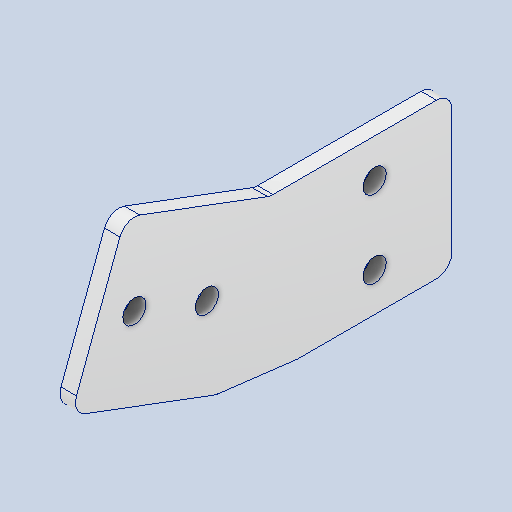
# Autodesk Inventor part: RZvector-v1-MP-Tr-F
Saved by Autodesk Inventor 2025.1 (Build 291241000, 241)
## iProperties
Created: 2024-03-17
Part Number: RZvector-v1-MP-Tr-F
Material: アルミニウム 6061
Document SubType Name: Modeling
Designer: haruy
Density: 2.7 g/cm^3
Appearance: アルミニウム - フラット
Mass: 1.7478 g
Surface Area: 21.5742 cm^2
Volume: 2.18475 cm^3
Author: haruy
Autodesk Inventor part; units mm, degrees
ref_plane "YZ Plane" through (0, 0, 0) normal (1, 0, 0) x (0, 1, 0)
ref_plane "XZ Plane" through (0, 0, 0) normal (0, 1, 0) x (-1, 0, 0)
ref_plane "XY Plane" through (0, 0, 0) normal (0, 0, 1) x (1, 0, 0)
derived "RZvector-arm-rotate-v1-Sketch-Base.ipt"
sketch "横から" plane through (0, 0, 0) normal (1, 0, 0) x (0, 1, 0)
  line L0 (0, 0) -> (0, -30.2937)
  line L1 (542.7807, -196.25) -> (0, -196.25)
  line L2 (628, -186.25) -> (24, -186.25)
  line L3 (24, -186.25) -> (24, -206.25)
  line L4 (24, -206.25) -> (628, -206.25)
  line L5 (628, -206.25) -> (628, -186.25)
  line L6 (138, -159.75) -> (123, -159.75)
  line L7 (123, -159.75) -> (123, -174.75)
  line L8 (123, -174.75) -> (138, -174.75)
  line L9 (138, -174.75) -> (138, -159.75)
  line L10 (0, 0) -> (0, -196.25)
  line L11 (138, -217.75) -> (123, -217.75)
  line L12 (123, -217.75) -> (123, -232.75)
  line L13 (123, -232.75) -> (138, -232.75)
  line L14 (138, -232.75) -> (138, -217.75)
  line L15 (0, 0) -> (0, -415.25)
  line L16 (54, -415.25) -> (34, -415.25)
  line L17 (34, -415.25) -> (34, -395.25)
  line L18 (34, -395.25) -> (54, -395.25)
  line L19 (54, -395.25) -> (54, -415.25)
  line L20 (134, -345.25) -> (64, -345.25)
  line L21 (64, -345.25) -> (64, -395.25)
  line L22 (64, -395.25) -> (134, -395.25)
  line L23 (134, -395.25) -> (134, -345.25)
  line L24 (136, -310.25) -> (134, -310.25)
  line L25 (134, -310.25) -> (134, -405.25)
  line L26 (134, -405.25) -> (136, -405.25)
  line L27 (136, -405.25) -> (136, -310.25)
  line L28 (136, -310.25) -> (146, -310.25)
  line L29 (146, -310.25) -> (146, -320.25)
  line L30 (146, -320.25) -> (136, -320.25)
  line L31 (136, -320.25) -> (136, -310.25)
  line L32 (146, -320.25) -> (54, -320.25)
  line L33 (54, -320.25) -> (54, -330.25)
  line L34 (54, -330.25) -> (146, -330.25)
  line L35 (146, -330.25) -> (146, -320.25)
  line L36 (0, -269) -> (385.3867, -269)
  line L37 (144, 54.75) -> (46, 54.75)
  line L38 (46, 54.75) -> (46, -139.45)
  line L39 (46, -139.45) -> (144, -139.45)
  line L40 (144, -139.45) -> (144, 54.75)
  circle A0 centre (95, 2.25) radius 95
  line L41 (176, -92.75) -> (156, -92.75)
  line L42 (156, -92.75) -> (156, -290.75)
  line L43 (156, -290.75) -> (176, -290.75)
  line L44 (176, -290.75) -> (176, -92.75)
  circle A1 centre (166, -269) radius 6
  circle A2 centre (166, -269) radius 22.5
  circle A3 centre (129.5351, -260.25) radius 15
  circle A4 centre (129.5351, -260.25) radius 6
  line L45 (138, -159.75) -> (153, -159.75)
  line L46 (153, -159.75) -> (153, -232.75)
  line L47 (153, -232.75) -> (138, -232.75)
  line L48 (138, -232.75) -> (138, -159.75)
  line L49 (123, -174.75) -> (153, -174.75)
  line L50 (153, -174.75) -> (153, -184.75)
  line L51 (153, -184.75) -> (123, -184.75)
  line L52 (123, -184.75) -> (123, -174.75)
  line L53 (123, -217.75) -> (153, -217.75)
  line L54 (153, -217.75) -> (153, -207.75)
  line L55 (153, -207.75) -> (123, -207.75)
  line L56 (123, -207.75) -> (123, -217.75)
  circle A5 centre (129.5351, -260.25) radius 18.75
  circle A6 centre (99.5351, -260.25) radius 15
  line L57 (136, -330.25) -> (146, -330.25)
  line L58 (146, -330.25) -> (146, -340.25)
  line L59 (146, -340.25) -> (136, -340.25)
  line L60 (136, -340.25) -> (136, -330.25)
  line L61 (54, -405.25) -> (56, -405.25)
  line L62 (56, -405.25) -> (56, -345.2512)
  line L63 (56, -345.2512) -> (54, -345.2512)
  line L64 (54, -345.2512) -> (54, -405.25)
  line L65 (56, -320.25) -> (64.683, -320.25)
  line L66 (54, -310.25) -> (64, -310.25)
  line L67 (64, -310.25) -> (64, -320.25)
  line L68 (64, -320.25) -> (54, -320.25)
  line L69 (54, -320.25) -> (54, -310.25)
  line L70 (54, -310.25) -> (44, -310.25)
  line L71 (44, -310.25) -> (44, -340.25)
  line L72 (44, -340.25) -> (54, -340.25)
  line L73 (54, -340.25) -> (54, -310.25)
  line L74 (34, -415.25) -> (54, -415.25)
  line L75 (54, -415.25) -> (54, -139.45)
  line L76 (54, -139.45) -> (34, -139.45)
  line L77 (34, -139.45) -> (34, -415.25)
  line L78 (628, -186.25) -> (659.5, -186.25)
  line L79 (659.5, -186.25) -> (659.5, -206.25)
  line L80 (659.5, -206.25) -> (628, -206.25)
  line L81 (628, -206.25) -> (628, -186.25)
  line L82 (54, -375.25) -> (34, -375.25)
  circle A7 centre (129.5351, -260.25) radius 12.5
  circle A8 centre (643.75, -167.5) radius 15.75
  line L83 (659.5, -186.25) -> (659.5, -167.5)
  line L84 (628, -186.25) -> (628, -167.5)
  line L85 (150.5, -293.5212) -> (150.5, -446.3995)
  line L86 (34, -395.25) -> (477, -395.25)
  line L87 (477, -395.25) -> (477, -375.25)
  line L88 (477, -375.25) -> (34, -375.25)
  line L89 (34, -375.25) -> (34, -395.25)
  line L90 (184, -375.25) -> (194, -375.25)
  line L91 (194, -375.25) -> (194, -365.25)
  line L92 (194, -365.25) -> (184, -365.25)
  line L93 (184, -365.25) -> (184, -375.25)
  line L94 (230, -365.25) -> (194, -365.25)
  line L95 (194, -365.25) -> (194, -399.25)
  line L96 (194, -399.25) -> (230, -399.25)
  line L97 (230, -399.25) -> (230, -365.25)
  line L98 (212, -365.25) -> (212, -399.25)
  line L99 (194, -365.25) -> (204, -365.25)
  line L100 (204, -365.25) -> (204, -395.25)
  line L101 (204, -395.25) -> (194, -395.25)
  line L102 (194, -395.25) -> (194, -365.25)
  circle A9 centre (496.8064, -373.1284) radius 1.5
  circle A10 centre (489.7967, -380.2604) radius 1.5
  circle A11 centre (219, -385.25) radius 1.5
  circle A12 centre (209, -385.25) radius 1.5
  line L103 (423, -49.3886) -> (335, -49.3886)
  line L104 (335, -49.3886) -> (335, -349.3886)
  line L105 (335, -349.3886) -> (423, -349.3886)
  line L106 (423, -349.3886) -> (423, -49.3886)
  line L107 (394, -349.3886) -> (364, -349.3886)
  line L108 (364, -349.3886) -> (364, -369.3886)
  line L109 (364, -369.3886) -> (394, -369.3886)
  line L110 (394, -369.3886) -> (394, -349.3886)
  line L111 (359, -365.25) -> (349, -365.25)
  line L112 (349, -365.25) -> (349, -375.25)
  line L113 (349, -375.25) -> (359, -375.25)
  line L114 (359, -375.25) -> (359, -365.25)
  line L115 (379, -349.3886) -> (379, -369.3886)
  line L116 (347, -375.25) -> (357, -375.25)
  circle A13 centre (472, -385.25) radius 1.5
  circle A14 centre (462, -385.25) radius 1.5
  line L117 (521, -49.3886) -> (433, -49.3886)
  line L118 (433, -49.3886) -> (433, -349.3886)
  line L119 (433, -349.3886) -> (521, -349.3886)
  line L120 (521, -349.3886) -> (521, -49.3886)
  line L121 (457, -375.25) -> (447, -375.25)
  line L122 (447, -375.25) -> (447, -365.25)
  line L123 (447, -365.25) -> (457, -365.25)
  line L124 (457, -365.25) -> (457, -375.25)
  line L125 (643.186, -209.9292) -> (479.1599, -376.8167)
  line L126 (479.1599, -376.8167) -> (493.4238, -390.836)
  line L127 (493.4238, -390.836) -> (657.4499, -223.9485)
  line L128 (657.4499, -223.9485) -> (643.186, -209.9292)
  line L129 (457, -375.25) -> (457, -395.25)
  line L130 (493.1793, -362.5528) -> (507.4432, -376.5721)
  line L131 (629.1667, -224.1931) -> (643.4306, -238.2124)
  line L132 (477, -375.25) -> (493.1793, -362.5528)
  line L133 (493.4238, -390.836) -> (477, -395.25)
  line L134 (230, -375.25) -> (220, -375.25)
  line L135 (220, -375.25) -> (220, -365.25)
  line L136 (220, -365.25) -> (230, -365.25)
  line L137 (230, -365.25) -> (230, -375.25)
  line L138 (230, -365.25) -> (65, -365.25)
  line L139 (65, -365.25) -> (65, -360.25)
  line L140 (65, -360.25) -> (230, -360.25)
  line L141 (230, -360.25) -> (230, -365.25)
  line L142 (220, -309.25) -> (65, -309.25)
  line L143 (65, -309.25) -> (65, -313.25)
  line L144 (65, -313.25) -> (220, -313.25)
  line L145 (220, -313.25) -> (220, -309.25)
  line L146 (65, -365.25) -> (70, -365.25)
  line L147 (70, -365.25) -> (70, -309.25)
  line L148 (70, -309.25) -> (65, -309.25)
  line L149 (65, -309.25) -> (65, -365.25)
  line L150 (239, -375.25) -> (239, -395.25)
  line L151 (130, -371.7504) -> (108.5351, -371.7504)
  line L152 (108.5351, -371.7504) -> (108.5351, -456.25)
  line L153 (108.5351, -456.25) -> (130, -456.25)
  line L154 (130, -456.25) -> (130, -371.7504)
  circle A15 centre (175, -269) radius 6
  line L155 (302.5611, -391.0338) -> (151.9649, -262.485)
  line L156 (151.9649, -262.485) -> (164.9496, -247.2732)
  line L157 (164.9496, -247.2732) -> (315.5458, -375.822)
  line L158 (315.5458, -375.822) -> (302.5611, -391.0338)
  circle A16 centre (427.4049, -391.1037) radius 95
  line L159 (900, 0) -> (900, -1750.1016)
  line L160 (525, -456.25) -> (0, -456.25)
  line L161 (0, -456.25) -> (0, -706.25)
  line L162 (0, -706.25) -> (525, -706.25)
  line L163 (525, -706.25) -> (525, -456.25)
  line L164 (286.9304, -332.3317) -> (437.1463, -460.5559)
  line L165 (437.1463, -460.5559) -> (497.5252, -389.8213)
  line L166 (497.5252, -389.8213) -> (347.3093, -261.5971)
  line L167 (347.3093, -261.5971) -> (286.9304, -332.3317)
  line L168 (659.5, -186.25) -> (668.5, -186.25)
  line L169 (668.5, -186.25) -> (668.5, -206.25)
  line L170 (668.5, -206.25) -> (659.5, -206.25)
  line L171 (659.5, -206.25) -> (659.5, -186.25)
  line L172 (224, -174.75) -> (194, -174.75)
  line L173 (194, -174.75) -> (194, -217.75)
  line L174 (194, -217.75) -> (224, -217.75)
  line L175 (224, -217.75) -> (224, -174.75)
  line L176 (605, -186.25) -> (605, -206.25)
  line L177 (242.3, -171.25) -> (226.4, -171.25)
  line L178 (226.4, -171.25) -> (226.4, -199.05)
  line L179 (226.4, -199.05) -> (242.3, -199.05)
  line L180 (242.3, -199.05) -> (242.3, -171.25)
  circle A17 centre (239.5, -196.25) radius 1.7
  circle A18 centre (229.2, -174.05) radius 1.7
  circle A19 centre (247.5, -196.25) radius 1.7
  line L181 (252.5, -186.25) -> (252.5, -206.25)
  line L182 (550.2984, 177.2044) -> (550.2984, -1079.3945)
  line L183 (477, -375.25) -> (590, -375.25)
  line L184 (590, -375.25) -> (590, -395.25)
  line L185 (590, -395.25) -> (477, -395.25)
  line L186 (477, -395.25) -> (477, -375.25)
  line L187 (590, -395.25) -> (578, -395.25)
  line L188 (578, -395.25) -> (578, -407.25)
  line L189 (578, -407.25) -> (590, -407.25)
  line L190 (590, -407.25) -> (590, -395.25)
  line L191 (239, -375.25) -> (229, -375.25)
  line L192 (229, -375.25) -> (229, -365.25)
  line L193 (229, -365.25) -> (239, -365.25)
  line L194 (239, -365.25) -> (239, -375.25)
  line L195 (245.8, -370.25) -> (224.6774, -352.1759)
  line L196 (224.6774, -352.1759) -> (236.9001, -337.8915)
  line L197 (236.9001, -337.8915) -> (258.0228, -355.9656)
  line L198 (258.0228, -355.9656) -> (245.8, -370.25)
  circle A20 centre (247.3784, -364.0987) radius 1.7
  circle A21 centre (237.2072, -341.8394) radius 1.7
  line L199 (239, -365.25) -> (249, -365.25)
  line L200 (249, -365.25) -> (249, -375.25)
  line L201 (249, -375.25) -> (239, -375.25)
  line L202 (239, -375.25) -> (239, -365.25)
  line L203 (249, -365.25) -> (224.6774, -365.25)
  line L204 (224.6774, -365.25) -> (224.6774, -355.25)
  line L205 (224.6774, -355.25) -> (249, -355.25)
  line L206 (249, -355.25) -> (249, -365.25)
  line L207 (224.6774, -365.25) -> (230, -365.25)
  line L208 (230, -365.25) -> (230, -375.25)
  line L209 (230, -375.25) -> (224.6774, -375.25)
  line L210 (224.6774, -375.25) -> (224.6774, -365.25)
  line L211 (224.6774, -352.1759) -> (224.6774, -355.25)
  line L212 (239, -368.75) -> (249, -368.75)
  line L213 (249, -368.75) -> (249, -371.75)
  line L214 (249, -371.75) -> (239, -371.75)
  line L215 (239, -371.75) -> (239, -368.75)
  line L216 (258.0228, -355.9656) -> (249, -375.25)
  line L217 (593.9382, -399.979) -> (576.2016, -378.5721)
  line L218 (576.2016, -378.5721) -> (590.6782, -366.5776)
  line L219 (590.6782, -366.5776) -> (608.4148, -387.9845)
  line L220 (608.4148, -387.9845) -> (593.9382, -399.979)
  circle A22 centre (596.5409, -394.1863) radius 1.7
  circle A23 centre (590.3086, -370.5201) radius 1.7
  line L221 (590, -407.25) -> (600, -407.25)
  line L222 (600, -407.25) -> (600, -397.25)
  line L223 (600, -397.25) -> (590, -397.25)
  line L224 (590, -397.25) -> (590, -407.25)
  line L225 (600, -397.25) -> (576.2016, -397.25)
  line L226 (576.2016, -397.25) -> (576.2016, -378.5721)
  line L227 (576.2016, -378.5721) -> (600, -378.5721)
  line L228 (600, -378.5721) -> (600, -397.25)
  line L229 (576.2016, -397.25) -> (578, -397.25)
  line L230 (578, -397.25) -> (578, -407.25)
  line L231 (578, -407.25) -> (576.2016, -407.25)
  line L232 (576.2016, -407.25) -> (576.2016, -397.25)
  line L233 (608.4148, -387.9845) -> (600, -407.25)
  line L234 (590, -375.25) -> (610, -375.25)
  line L235 (610, -375.25) -> (610, -395.25)
  line L236 (610, -395.25) -> (590, -395.25)
  line L237 (590, -395.25) -> (590, -375.25)
  line L238 (648.5, -186.25) -> (648.5, -206.25)
  line L239 (667.9052, -217.2444) -> (610, -371.75)
  line L240 (610, -371.75) -> (591.272, -364.7312)
  line L241 (591.272, -364.7312) -> (649.1773, -210.2256)
  line L242 (649.1773, -210.2256) -> (667.9052, -217.2444)
  line L243 (660.8864, -235.9723) -> (642.1585, -228.9535)
  line L244 (617.0188, -353.022) -> (598.2909, -346.0032)
  line L245 (610, -371.75) -> (610, -375.25)
  line L246 (591.272, -364.7312) -> (590, -375.25)
  circle A24 centre (605, -385.25) radius 1.5
  circle A25 centre (595, -385.25) radius 1.5
  circle A26 centre (605.9001, -354.1946) radius 1.5
  circle A27 centre (602.3907, -363.5586) radius 1.5
  point P0 (166, -92.75)
  point P1 (204, -375.25)
  point P2 (394, -359.3886)
  point P3 (643.75, -206.25)
  point P4 (247.4615, -346.9286)
  point P5 (590, -395.2259)
  point P6 (591.677, -397.25)
  point P7 (600, -395.25)
  point P8 (591.0016, -366.9679)
  point P9 (597.8637, -375.25)
  point P10 (590.02, -395.25)
  point P11 (599.6458, -395.25)
  point P12 (590, -395.2259)
  point P13 (580.2112, -375.25)
  point P14 (597.2319, -397.25)
  point P15 (600, -394.9565)
  point P16 (600, -395.25)
  dimension "d2" = 3
  dimension "d3" = 3
  dimension "d4" = 3
  dimension "d5" = 3
  dimension "d6" = 5
  dimension "d7" = 10
  dimension "d8" = 10
  dimension "d9" = 10
  dimension "d14" = 10
  dimension "d18" = 3
  dimension "d19" = 3
  dimension "d20" = 5
  dimension "d21" = 10
  dimension "d22" = 10
  dimension "d23" = 10
  dimension "d24" = 10
  dimension "d25" = 5
  dimension "d26" = 10
  dimension "d27" = 3
  dimension "d28" = 3
  dimension "d29" = 5
  dimension "d30" = 10
  dimension "d31" = 10
  dimension "d32" = 10
  dimension "d33" = 3
  dimension "d34" = 3
  dimension "d35" = 5
  dimension "d36" = 10
  dimension "d37" = 10
  dimension "d38" = 10
  measures "d2" diameter of A9
  measures "d3" diameter of A10
  measures "d4" diameter of A11
  measures "d5" diameter of A12
  measures "d6" distance from line of A12.centre L100
  measures "d7" distance of A11.centre A12.centre
  measures "d8" distance from line of A12.centre L88
  measures "d9" distance from line of L88 A11.centre
  measures "d14" distance of A10.centre A9.centre
  measures "d18" diameter of A13
  measures "d19" diameter of A14
  measures "d20" distance from line of A13.centre L87
  measures "d21" distance of A14.centre A13.centre
  measures "d22" distance from line of A14.centre L86
  measures "d23" distance from line of A13.centre L86
  measures "d24" distance from line of A9.centre L127
  measures "d25" distance from line of L126 A10.centre
  measures "d26" distance from line of A10.centre L127
  measures "d27" diameter of A24
  measures "d28" diameter of A25
  measures "d29" distance from line of A24.centre L235
  measures "d30" distance of A24.centre A25.centre
  measures "d31" distance from line of A24.centre L236
  measures "d32" distance from line of L236 A25.centre
  measures "d33" diameter of A26
  measures "d34" diameter of A27
  measures "d35" distance from line of A26.centre L244
  measures "d36" distance of A27.centre A26.centre
  measures "d37" distance from line of A26.centre L241
  measures "d38" distance from line of A27.centre L241
extrude "押し出し1" add sketch "横から" along normal blind 2 contours L244 L239 L240 L241 | L240 L245 L234 L219 L246 | L234 L219 A24 L220 L228 L227 L184 | L246 A23 L219 L234 | L227 L228 L220 L236 A22 L217 L184 | L234 L235 L236 L233 L219 A24 | L246 A23 | L217 L236 L184 | L228 L236 L220 | L220 L233 L236 L228 | A22 L236 picked at (591.0527, -370.87) picked at (596.0137, -394.5304)
fillet "フィレット2" radius 2 7 edges at (1, 610, -371.75) (1, 617.0188, -353.022) (1, 598.2909, -346.0032) (1, 591.272, -364.7312) (1, 590, -375.25) (1, 610, -395.25) (1, 590, -395.25)
